shankHolder.5in_v21 (Autodesk Fusion 360 design; units mm, degrees)
Autodesk Fusion 360 part; units mm, degrees
note: some values were not read from the file. Set by a fixed rule: the direction of a hole.
sketch "Sketch1" plane through (0, 0, 0) normal (0, 0, 1) x (1, 0, 0)
  circle A0 centre (0, 0) radius 18.2563
  circle A1 centre (0, 0) radius 15.0812 construction
  line L0 (0, 0) -> (0, 18.2563) construction
  line L1 (3.5929, -6.223) -> (7.1857, 0)
  line L2 (7.1857, 0) -> (3.5929, 6.223)
  line L3 (3.5929, 6.223) -> (-3.5929, 6.223)
  line L4 (-3.5929, 6.223) -> (-7.1857, 0)
  line L5 (-7.1857, 0) -> (-3.5929, -6.223)
  line L6 (-3.5929, -6.223) -> (3.5929, -6.223)
  point P0 (0, 15.0812)
  dimension "d1" = 36.5125
  dimension "d2" = 30.1625
  dimension "d3" = 6.223
  constraint coincident A0.centre A1.centre
  constraint coincident A0 L0.end
  constraint vertical L0
  constraint coincident L0 P0
  constraint coincident A1 P0
  constraint horizontal L6
  measures "d1" diameter of A0
  measures "d2" diameter of A1
  measures "d3" distance of A0.centre L6
extrude "Extrude1" add sketch "Sketch1" along normal blind 6.35
extrude "Extrude2" add sketch "Sketch1" along normal blind 19.05 contours L1 L2 L3 L4 L5 L6
hole "Hole1" at (0, 15.0812, 0) direction (0, 0, 1) diameter 2.7686 depth 6.35 tip angle 118
thread "Thread1" "ANSI Unified Screw Threads 0.138(#6) 6-32 UNC 2B"
pattern_circular "C-Pattern1" count 3 over 360 about axis through (0, 0, 0) along (0, 0, 1) of "Hole1"
fillet "Fillet1" radius 1.5875 6 edges at (3.5929, -6.223, 12.7) (-3.5929, -6.223, 12.7) (-7.1857, 0, 12.7) (-3.5929, 6.223, 12.7) (3.5929, 6.223, 12.7) (7.1857, 0, 12.7)
equation "d4 = 0.25 in"
equation "d6 = d4 + shankLength"
equation "d14 = ( 1 / 16 ) * 1 in"
equation "shankLength = 0.5 in"
